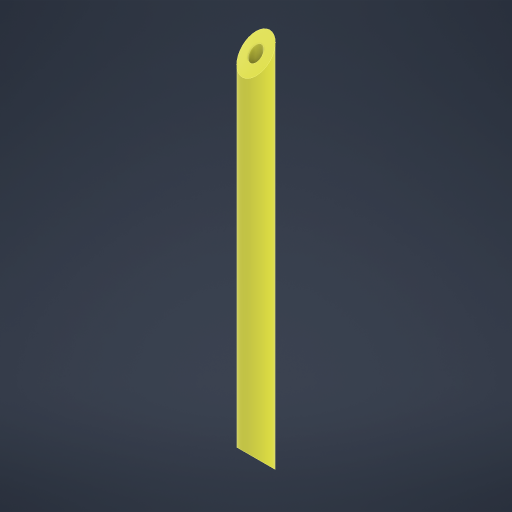
# Autodesk Inventor part: BUMP_004_Noodle2
Saved by Autodesk Inventor 2024.2 (Build 282272000, 272)
## iProperties
Created: 2024-08-07
Part Number: BUMP_004_Noodle2
Material: Pool Noodle
Document SubType Name: Modeling
Designer: Bryan
Density: 0.0276799 g/cm^3
Appearance: Yellow
Mass: 67.3314 g
Surface Area: 2629.05 cm^2
Volume: 2432.5 cm^3
Author: Bryan
Autodesk Inventor part; units mm, degrees
ref_plane "XZ Plane" through (0, 0, 0) normal (0, 1, 0) x (-1, 0, 0)
ref_plane "XY Plane" through (0, 0, 0) normal (0, 0, 1) x (1, 0, 0)
sketch "Sketch1" plane through (0, 0, 0) normal (0, 1, 0) x (-1, 0, 0)
  circle A0 centre (0, 0) radius 12.7
  circle A1 centre (0, 0) radius 31.75
  dimension "d0" = 63.5
  dimension "d1" = 25.4
  constraints: 2 centre point, 2 coincident
  measures "d0" diameter of A1
  measures "d1" diameter of A0
extrude "Extrusion1" add sketch "Sketch1" along normal blind 876.3
ref_plane "Work Plane1" through (-31.75, 0, 0) normal (1, 0, 0) x (0, 1, 0)
sketch "Sketch2" plane through (-31.75, 0, 0) normal (1, 0, 0) x (0, 1, 0)
  line L0 (876.3, -31.75) -> (876.3, 31.75) projected
  line L1 (0, -31.75) -> (0, 31.75) projected
  line L2 (0, -31.75) -> (63.5, 31.75)
  line L3 (0, 31.75) -> (876.3, 31.75) projected
  line L4 (876.3, -31.75) -> (812.8, 31.75)
  dimension "d5" = 45
  dimension "d6" = 45
  constraints: 4 end point, 2 point on line
  measures "d5" angle of L1 L2
  measures "d6" angle of L3 L4
extrude "Extrusion2" cut sketch "Sketch2" along normal blind 977.9
body "Solid1"
